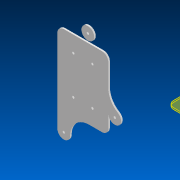
# Autodesk Inventor part: Brain Mount
Saved by Autodesk Inventor 2022 (Build 260153000, 153)
## iProperties
Created: 2022-04-13
Part Number: Brain Mount
Material: Generic
Document SubType Name: Modeling
Designer: score_nygvs6w
Density: 1 g/cm^3
Appearance: Default
Author: score_nygvs6w
Autodesk Inventor part; units mm, degrees
ref_plane "YZ Plane" through (0, 0, 0) normal (1, 0, 0) x (0, 1, 0)
ref_plane "XZ Plane" through (0, 0, 0) normal (0, 1, 0) x (-1, 0, 0)
ref_plane "XY Plane" through (0, 0, 0) normal (0, 0, 1) x (1, 0, 0)
sketch "Sketch1" plane through (0, 0, 0) normal (0, 0, 1) x (1, 0, 0)
  line L0 (19.05, 38.1) -> (-19.05, 38.1) construction
  line L1 (-19.05, 38.1) -> (-19.05, -38.1) construction
  line L2 (-19.05, -38.1) -> (19.05, -38.1) construction
  line L3 (19.05, -38.1) -> (19.05, 38.1) construction
  line L4 (19.05, 38.1) -> (-19.05, -38.1) construction
  line L5 (-19.05, 38.1) -> (19.05, -38.1) construction
  line L6 (-50.8, -69.85) -> (38.1, -69.85)
  line L7 (50.8, -57.15) -> (50.8, 57.15)
  line L8 (38.1, 69.85) -> (-38.1, 69.85)
  line L9 (-50.8, 57.15) -> (-50.8, -69.85)
  line L10 (-50.8, -69.85) -> (50.8, 69.85) construction
  line L11 (50.8, -69.85) -> (-50.8, 69.85) construction
  circle A0 centre (18.4474, 77.2895) radius 12.7
  circle A1 centre (63.5, -31.75) radius 12.7
  circle A2 centre (-38.1, -107.95) radius 12.7
  arc A3 (-6.4019, 69.85) -> (6.0228, 79.9198) centre (-6.4019, 82.55) ccw
  arc A4 (50.8, -6.35) -> (63.5, -19.05) centre (63.5, -6.35) ccw
  arc A5 (63.5, -44.45) -> (50.8, -57.15) centre (63.5, -57.15) ccw
  arc A6 (12.7, -69.85) -> (-25.4, -107.95) centre (12.7, -107.95) ccw
  line L12 (-50.8, -107.95) -> (-50.8, -69.85)
  arc A7 (38.1, -69.85) -> (50.8, -57.15) centre (38.1, -57.15) ccw
  arc A8 (50.8, 57.15) -> (38.1, 69.85) centre (38.1, 57.15) ccw
  arc A9 (-38.1, 69.85) -> (-50.8, 57.15) centre (-38.1, 57.15) ccw
  arc A10 (19.9641, 75.8806) -> (17.0385, 78.8062) centre (18.4474, 77.2895) ccw
  arc A11 (50.8, 57.15) -> (18.7582, 89.9857) centre (17.9544, 57.15) ccw
  point P0 (0, 0)
  point P1 (-38.1, -69.85)
  point P2 (-50.8, -78.4346)
  point P3 (50.8, -31.75)
  point P4 (8.1546, 69.85)
  point P5 (28.7403, 69.85)
  dimension "d0" = 38.1
  dimension "d1" = 76.2
  dimension "d2" = 31.75
  dimension "d3" = 31.75
  dimension "d13" = 25.4
  dimension "d20" = 12.7
  dimension "d21" = 76.2
  dimension "d22" = 38.1
  dimension "d23" = 32.8456
  constraints: 26 end point, 25 point on circle, 18 tangent, 12 centre point, 10 point on line, 8 coincident, 7 equal radius, 4 midpoint, 4 parallel, 2 horizontal, 2 perpendicular, 1 horizontal alignment, 1 vertical, 4 other
  measures "d0" distance of L2.end L1.end
  measures "d1" distance of L1.end L0.end
  measures "d2" distance between parallel lines of L0 L8
  measures "d3" distance between parallel lines of L9 L1
  measures "d13" diameter of A0
  measures "d20" radius of A7
  measures "d21" vertical distance of point (-38.1, -107.95) point (63.5, -31.75)
  measures "d22" distance from line of L6 point (-38.1, -107.95)
  measures "d23" radius of A11
extrude "Extrusion1" add sketch "Sketch1" along normal blind 3.175
hole "Hole1" at (-19.05, 38.1, 0) at (19.05, 38.1, 0) at (19.05, -38.1, 0) at (-19.05, -38.1, 0) at (-38.1, -107.95, 0) at (63.5, -31.75, 0) at (18.4474, 77.2895, 0) direction (0, 0, 1) diameter 4.572 end through all
body "Solid1"
